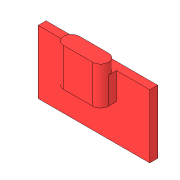
# Autodesk Inventor part: ‎BOB-15100‎ USB C Breakout
Saved by Autodesk Inventor 2018.3 (Build 223284000, 284)
## iProperties
Created: 2018-12-11
Part Number: ‎BOB-15100‎ USB C Breakout
Material: PBT Plastic
Document SubType Name: Modeling
Designer: tei06398
Mass: 0.862161 g
Surface Area: 8.09375 cm^2
Volume: 0.658138 cm^3
Density: 1.31 g/cm^3
Appearance: Smooth - White
Author: tei06398
Autodesk Inventor part; units mm, degrees
ref_plane "YZ Plane" through (0, 0, 0) normal (1, 0, 0) x (0, 1, 0)
ref_plane "XZ Plane" through (0, 0, 0) normal (0, 1, 0) x (-1, 0, 0)
ref_plane "XY Plane" through (0, 0, 0) normal (0, 0, 1) x (1, 0, 0)
sketch "Sketch1" plane through (0, 0, 0) normal (0, 0, 1) x (1, 0, 0)
  line L0 (0, 0) -> (22.352, 0)
  line L1 (22.352, 0) -> (22.352, 12.7)
  line L2 (22.352, 12.7) -> (0, 12.7)
  line L3 (0, 12.7) -> (0, 0)
  dimension "d0" = 22.352
  dimension "d1" = 12.7
  constraints: 8 end point, 2 parallel, 1 horizontal, 1 perpendicular
  measures "d0" distance of L2.end L1.end
  measures "d1" distance of L1.end L0.end
extrude "Extrusion1" add sketch "Sketch1" against normal blind 1.5875
sketch "Sketch2" plane through (0, 0, 0) normal (0, 0, 1) x (1, 0, 0)
  line L0 (22.352, 0) -> (22.352, 12.7) projected
  line L1 (6.6675, 14.9342) -> (15.6845, 14.9342)
  line L2 (15.6845, 14.9342) -> (15.6845, 7.3142)
  line L3 (15.6845, 7.3142) -> (6.6675, 7.3142)
  line L4 (6.6675, 7.3142) -> (6.6675, 14.9342)
  dimension "d8" = 9.017
  dimension "d9" = 7.62
  dimension "d10" = 6.6675
  constraints: 8 end point, 2 parallel, 1 horizontal, 1 perpendicular
  measures "d8" distance of L1.start L1.end
  measures "d9" distance of L1.end L2.end
  measures "d10" distance between parallel lines of L0 L2
extrude "Extrusion2" add sketch "Sketch2" along normal blind 3.175
fillet "Fillet1" radius 1.5875 4 edges at (15.6845, 11.1242, 3.175) (15.6845, 13.8171, 0) (6.6675, 11.1242, 3.175) (6.6675, 13.8171, 0)
body "Solid1"
